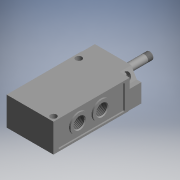
# Autodesk Inventor part: 6211 MFH-5-1/4
Saved by Autodesk Inventor 2017.3 (Build 213256000, 256)
## iProperties
Part Number: 6211 MFH-5-1/4
Material: Generic
Catalog Web Link: www.cadenas.de
Description: MFH-Solenoid valve
Vendor: FESTO
Document SubType Name: Modeling
Designer: partserver
Manufacturer: FESTO
Mass: 290 g
Surface Area: 238.767 cm^2
Volume: 130.921 cm^3
Density: 1 g/cm^3
Appearance: PSOLRGB-175-175-175
Category: PARTsolutions
Company: FESTO
Title: 6211 MFH-5-1/4
Author: Cadenas PARTsolutions
Comments: Solenoid valve
PSOL_IDENT_0: {$CADENAS_DATA\23d-libs\festo\parts\m\mfh\mfh.prj},166 {VTYP=3D},{NB=6211 MFH-5-1/4},{LINA=6211 MFH-
PSOL_IDENT_1: 5-1/4},{NN=MFH},{DATE=30.03.2021 15:09:58},{GEOMDATE=15.12.2020 07:36:11},{VERSION=},{LINEID=180},{W
PSOL_IDENT_2: BVAR=},{WBNUMERIC=}  {NB=6211 MFH-5-1/4},{LINA=6211 MFH-5-1/4},{KT=DUMMY},{TNR=6211},{TYP=MFH-5-1/4}
PSOL_IDENT_3: ,{INFO=},{S=0.000},{VERS=6.000},{AW=0.000},{A=30.000},{A1=49.600},{A2=14.000},{A3=12.500},{A4=19.600
PSOL_IDENT_4: },{A5=12.000},{A6=20.000},{A7=28.000},{A8=30.000},{A9=7.820},{A10=13.700},{A11=0.000},{A12=0.000},{A
PSOL_IDENT_5: 13=0.000},{A14=0.000},{A15=0.000},{A16=0.000},{A17=0.000},{L01=80.000},{EX=0.000},{EX1=0.000},{EX2=0
PSOL_IDENT_6: .000},{EX3=0.000},{EX4=0.000},{EX5=0.000},{EX6=0.000},{EXW=0.000},{L0=0.000},{L03=0.000},{B0=0.000},
PSOL_IDENT_7: {B=0.000},{B1=30.400},{B2=0.000},{B3=5.000},{B4=4.000},{B5=0.000},{B6=0.000},{B7=0.000},{B8=0.000},{
PSOL_IDENT_8: B9=0.000},{D1=G1/4},{D1P=13.157},{KDR1=11.445},{D2=M5},{D2P=5.000},{KDRD2=4.134},{D3=6.500},{D3P=0.0
PSOL_IDENT_9: 00},{KDRD3=0.000},{D4=0.000},{D5=0.000},{D6=0.000},{H1=128.000},{H2=143.000},{H3=12.000},{H4=24.000}
PSOL_IDENT_10: ,{H5=28.000},{H6=9.500},{H7=128.000},{H8=94.000},{H9=8.000},{H10=0.000},{H11=0.000},{H12=0.000},{H13=
PSOL_IDENT_11: 0.000},{H14=0.000},{H15=0.000},{H16=0.000},{H17=0.000},{H18=0.000},{H19=0.000},{H20=0.000},{H21=0.00
PSOL_IDENT_12: 0},{H22=0.000},{H23=0.000},{H24=0.000},{H25=0.000},{HR1=5.000},{HR2=72.000},{HR3=0.000},{HR4=0.000},
PSOL_IDENT_13: {L21=40.000},{K=0.000},{L1=50.000},{L2=74.000},{L3=0.000},{L4=0.000},{L5=0.000},{L6=0.000},{L8=0.000
PSOL_IDENT_14: },{L9=0.000},{L10=0.000},{L11=0.000},{L12=0.000},{PSTOL=0.1},{ZZZ=0.000},{V=0.000},{B00=0.000},{B01=
PSOL_IDENT_15: 0.000},{B02=0.000},{B03=0.000},{L02=0.000},{CNSMASSEXACT=0.290},{L7=MIN},{EOLDATE=}
NB: 6211 MFH-5-1/4
NN: MFH
NT: Solenoid valve
NBSYN: $TNR. $TYP.
LINA: 6211 MFH-5-1/4
CATALOG: Festo
OFFICIAL_STANDARD_NUMBERS: ISO 1, ISO 2, ISO 3, ISO 4
TNR: 6211
TYP: MFH-5-1/4
B: 0
B1: 30.4
B2: 0
B3: 5
B4: 4
B5: 0
B6: 0
B7: 0
B8: 0
B9: 0
D1: G1/4
D2: M5
D3: 6.5
D4: 0
D5: 0
D6: 0
H1: 128
H2: 143
H3: 12
H4: 24
H5: 28
H6: 9.5
H7: 128
H8: 94
H9: 8
H10: 0
H11: 0
H12: 0
H13: 0
H14: 0
H15: 0
H16: 0
H17: 0
H18: 0
H19: 0
H20: 0
H21: 0
H22: 0
H23: 0
H24: 0
H25: 0
HR1: 5
HR2: 72
HR3: 0
HR4: 0
L21: 40
L1: 50
L2: 74
L3: 0
L4: 0
L5: 0
L6: 0
L8: 0
L9: 0
L10: 0
L11: 0
L12: 0
CNSMASSEXACT: 0.29
SUPPLIER: FESTO
ARTICLENO: 6211 MFH-5-1/4
BOMINFO: 6211 MFH-5-1/4
CREATOR: CADENAS GmbH
Autodesk Inventor part; units mm, degrees
ref_plane "YZ Plane" through (0, 0, 0) normal (1, 0, 0) x (0, 1, 0)
ref_plane "XZ Plane" through (0, 0, 0) normal (0, 1, 0) x (-1, 0, 0)
ref_plane "XY Plane" through (0, 0, 0) normal (0, 0, 1) x (1, 0, 0)
sketch "Skizze_1" plane through (0, 0, 0) normal (0, 0, 1) x (1, 0, 0)
  line L0 (-25, 94) -> (-25, 0)
  line L1 (-25, 0) -> (25, 0)
  line L2 (25, 0) -> (25, 94)
  line L3 (25, 94) -> (-25, 94)
  constraints: 8 end point
extrude "Extrusion1" add sketch "Skizze_1" along normal mid plane 30.4
sketch "Sketch_1" plane through (0, 94, 0) normal (0, 1, 0) x (1, 0, 0)
  line L0 (-34.8, -25) -> (34.8, -25)
  line L1 (34.8, -25) -> (34.8, 25)
  line L2 (34.8, 25) -> (-34.8, 25)
  line L3 (-34.8, 25) -> (-34.8, -25)
  line L4 (-24.8, -15) -> (24.8, -15)
  line L5 (24.8, -15) -> (24.8, 15)
  line L6 (24.8, 15) -> (-24.8, 15)
  line L7 (-24.8, 15) -> (-24.8, -15)
  constraints: 16 end point
extrude "Extrusion2" cut sketch "Sketch_1" against normal blind 14
sketch "Sketch_9" plane through (0, 94, 0) normal (0, 1, 0) x (1, 0, 0)
  line L0 (-24.8, 4.6077) -> (-19.9719, 4.6077)
  line L1 (-19.9719, 4.6077) -> (-13.9719, 15)
  line L2 (-13.9719, 15) -> (-24.8, 15)
  line L3 (-24.8, 15) -> (-24.8, 4.6077)
  constraints: 8 end point
extrude "Extrusion3" cut sketch "Sketch_9" against normal blind 12.5
sketch "Sketch_10" plane through (0, 0, 10) normal (0, 0, 1) x (1, 0, 0)
  line L0 (-14, 92.8708) -> (-14, 94)
  line L1 (-14, 94) -> (-10.3, 94)
  line L2 (-10.3, 94) -> (-10.3, 89.4)
  line L3 (-10.3, 89.4) -> (-10.5, 89.4)
  line L4 (-10.5, 89.4) -> (-10.5, 92.9)
  arc A0 (-10.5, 92.9) -> (-11, 93.4) centre (-11, 92.9) ccw
  line L5 (-11, 93.4) -> (-12.025, 93.4)
  line L6 (-12.025, 93.4) -> (-14, 92.8708)
  line L7 (-14, 92.8708) -> (-14, 94)
  constraints: 16 end point, 2 point on circle, 1 centre point
revolve "Revolution1" cut sketch "Sketch_10" angle 360 about axis through (-14, 92.8708, 10) along (0, -1, 0)
sketch "Sketch_11" plane through (0, 0, -10) normal (0, 0, 1) x (1, 0, 0)
  line L0 (14, 92.8708) -> (14, 94)
  line L1 (14, 94) -> (17.7, 94)
  line L2 (17.7, 94) -> (17.7, 89.4)
  line L3 (17.7, 89.4) -> (17.5, 89.4)
  line L4 (17.5, 89.4) -> (17.5, 92.9)
  arc A0 (17.5, 92.9) -> (17, 93.4) centre (17, 92.9) ccw
  line L5 (17, 93.4) -> (15.975, 93.4)
  line L6 (15.975, 93.4) -> (14, 92.8708)
  line L7 (14, 92.8708) -> (14, 94)
  constraints: 16 end point, 2 point on circle, 1 centre point
revolve "Revolution2" cut sketch "Sketch_11" angle 360 about axis through (14, 92.8708, -10) along (0, -1, 0)
sketch "Sketch_12" plane through (0, 94, 0) normal (0, 1, 0) x (1, 0, 0)
  arc A0 (-15.1708, -8.8679) -> (-15.5658, -9.5521) centre (-15.3683, -9.21) ccw
  line L0 (-15.5658, -9.5521) -> (-15.54, -9.567)
  arc A1 (-15.54, -10.433) -> (-15.54, -9.567) centre (-15.79, -10) ccw
  line L1 (-15.54, -10.433) -> (-15.5658, -10.4479)
  arc A2 (-15.5658, -10.4479) -> (-15.1708, -11.1321) centre (-15.3683, -10.79) ccw
  line L2 (-15.1708, -11.1321) -> (-15.145, -11.1172)
  arc A3 (-14.395, -11.5502) -> (-15.145, -11.1172) centre (-14.895, -11.5502) ccw
  line L3 (-14.395, -11.5502) -> (-14.395, -11.58)
  arc A4 (-14.395, -11.58) -> (-13.605, -11.58) centre (-14, -11.58) ccw
  line L4 (-13.605, -11.58) -> (-13.605, -11.5502)
  arc A5 (-12.855, -11.1172) -> (-13.605, -11.5502) centre (-13.105, -11.5502) ccw
  line L5 (-12.855, -11.1172) -> (-12.8292, -11.1321)
  arc A6 (-12.8292, -11.1321) -> (-12.4342, -10.4479) centre (-12.6317, -10.79) ccw
  line L6 (-12.4342, -10.4479) -> (-12.46, -10.433)
  arc A7 (-12.46, -9.567) -> (-12.46, -10.433) centre (-12.21, -10) ccw
  line L7 (-12.46, -9.567) -> (-12.4342, -9.5521)
  arc A8 (-12.4342, -9.5521) -> (-12.8292, -8.8679) centre (-12.6317, -9.21) ccw
  line L8 (-12.8292, -8.8679) -> (-12.855, -8.8828)
  arc A9 (-13.605, -8.4498) -> (-12.855, -8.8828) centre (-13.105, -8.4498) ccw
  line L9 (-13.605, -8.4498) -> (-13.605, -8.42)
  arc A10 (-13.605, -8.42) -> (-14.395, -8.42) centre (-14, -8.42) ccw
  line L10 (-14.395, -8.42) -> (-14.395, -8.4498)
  arc A11 (-15.145, -8.8828) -> (-14.395, -8.4498) centre (-14.895, -8.4498) ccw
  line L11 (-15.145, -8.8828) -> (-15.1708, -8.8679)
  constraints: 24 end point, 24 point on circle, 12 centre point
extrude "Extrusion4" cut sketch "Sketch_12" against normal blind 2.4
sketch "Sketch_13" plane through (0, 94, 0) normal (0, 1, 0) x (1, 0, 0)
  arc A0 (12.4342, 9.5521) -> (12.8292, 8.8679) centre (12.6317, 9.21) ccw
  line L0 (12.8292, 8.8679) -> (12.855, 8.8828)
  arc A1 (13.605, 8.4498) -> (12.855, 8.8828) centre (13.105, 8.4498) ccw
  line L1 (13.605, 8.4498) -> (13.605, 8.42)
  arc A2 (13.605, 8.42) -> (14.395, 8.42) centre (14, 8.42) ccw
  line L2 (14.395, 8.42) -> (14.395, 8.4498)
  arc A3 (15.145, 8.8828) -> (14.395, 8.4498) centre (14.895, 8.4498) ccw
  line L3 (15.145, 8.8828) -> (15.1708, 8.8679)
  arc A4 (15.1708, 8.8679) -> (15.5658, 9.5521) centre (15.3683, 9.21) ccw
  line L4 (15.5658, 9.5521) -> (15.54, 9.567)
  arc A5 (15.54, 10.433) -> (15.54, 9.567) centre (15.79, 10) ccw
  line L5 (15.54, 10.433) -> (15.5658, 10.4479)
  arc A6 (15.5658, 10.4479) -> (15.1708, 11.1321) centre (15.3683, 10.79) ccw
  line L6 (15.1708, 11.1321) -> (15.145, 11.1172)
  arc A7 (14.395, 11.5502) -> (15.145, 11.1172) centre (14.895, 11.5502) ccw
  line L7 (14.395, 11.5502) -> (14.395, 11.58)
  arc A8 (14.395, 11.58) -> (13.605, 11.58) centre (14, 11.58) ccw
  line L8 (13.605, 11.58) -> (13.605, 11.5502)
  arc A9 (12.855, 11.1172) -> (13.605, 11.5502) centre (13.105, 11.5502) ccw
  line L9 (12.855, 11.1172) -> (12.8292, 11.1321)
  arc A10 (12.8292, 11.1321) -> (12.4342, 10.4479) centre (12.6317, 10.79) ccw
  line L10 (12.4342, 10.4479) -> (12.46, 10.433)
  arc A11 (12.46, 9.567) -> (12.46, 10.433) centre (12.21, 10) ccw
  line L11 (12.46, 9.567) -> (12.4342, 9.5521)
  constraints: 24 end point, 24 point on circle, 12 centre point
extrude "Extrusion5" cut sketch "Sketch_13" against normal blind 2.4
sketch "Skizze_3" plane through (0, 0, 0) normal (0, 0, 1) x (1, 0, 0)
  circle A0 centre (-20, 5) radius 3.25
  constraints: 1 centre point
extrude "Extrusion6" cut sketch "Skizze_3" along normal mid plane 60.8
sketch "Skizze_13" plane through (0, 0, 0) normal (0, 0, 1) x (1, 0, 0)
  circle A0 centre (20, 72) radius 3.25
  constraints: 1 centre point
extrude "Extrusion7" cut sketch "Skizze_13" along normal mid plane 60.8
sketch "Skizze_7" plane through (-25, 0, -15.2) normal (-1, 0, 0) x (0, 0, 1)
  line L0 (2.0064, 52) -> (2.0064, 6.5664)
  arc A0 (2.0064, 6.5664) -> (3.0096, 5.5632) centre (3.0096, 6.5664) ccw
  line L1 (3.0096, 5.5632) -> (27.3904, 5.5632)
  arc A1 (27.3904, 5.5632) -> (28.3936, 6.5664) centre (27.3904, 6.5664) ccw
  line L2 (28.3936, 6.5664) -> (28.3936, 52)
  line L3 (28.3936, 52) -> (2.0064, 52)
  constraints: 8 end point, 4 point on circle, 2 centre point
extrude "Extrusion8" cut sketch "Skizze_7" along normal mid plane 3
sketch "Sketch_3" plane through (-25, 0, -15.2) normal (-1, 0, 0) x (0, 0, 1)
  line L0 (2.0064, 74.9904) -> (2.0064, 52)
  line L1 (2.0064, 52) -> (28.3936, 52)
  line L2 (28.3936, 52) -> (28.3936, 74.9904)
  arc A0 (28.3936, 74.9904) -> (27.3904, 75.9936) centre (27.3904, 74.9904) ccw
  line L3 (27.3904, 75.9936) -> (3.0096, 75.9936)
  arc A1 (3.0096, 75.9936) -> (2.0064, 74.9904) centre (3.0096, 74.9904) ccw
  constraints: 8 end point, 4 point on circle, 2 centre point
extrude "Extrusion9" cut sketch "Sketch_3" against normal blind 1.5
sketch "Skizze_15" plane through (-25, 0, -15.2) normal (-1, 0, 0) x (0, 0, 1)
  circle A0 centre (15.2, 52) radius 9.8678
  constraints: 1 centre point
extrude "Extrusion10" add sketch "Skizze_15" against normal blind 1.5
sketch "Skizze_6" plane through (0, 0, 0) normal (0, 0, 1) x (1, 0, 0)
  line L0 (-12.5, 52) -> (-25, 52)
  line L1 (-25, 52) -> (-25, 58.5785)
  line L2 (-25, 58.5785) -> (-24.144, 57.7225)
  line L3 (-24.144, 57.7225) -> (-12.5, 57.7225)
  line L4 (-12.5, 57.7225) -> (-12.5, 52)
  line L5 (-12.5, 52) -> (-25, 52)
  constraints: 12 end point
revolve "Revolution3" cut sketch "Skizze_6" angle 360 about axis through (-12.5, 52, 0) along (1, 0, 0)
thread "Thread1" size "G13.157x1.337" designation "G 1/4" standard "ISO Pipe Threads" full length
sketch "Skizze_16" plane through (-25, 0, 15.2) normal (-1, 0, 0) x (0, 1, 0)
  circle A0 centre (28, 15.2) radius 9.8678
  constraints: 1 centre point
extrude "Extrusion11" add sketch "Skizze_16" against normal blind 2
sketch "Skizze_8" plane through (0, 0, 0) normal (0, 0, 1) x (1, 0, 0)
  line L0 (-12.5, 28) -> (-25, 28)
  line L1 (-25, 28) -> (-25, 34.5785)
  line L2 (-25, 34.5785) -> (-24.144, 33.7225)
  line L3 (-24.144, 33.7225) -> (-12.5, 33.7225)
  line L4 (-12.5, 33.7225) -> (-12.5, 28)
  line L5 (-12.5, 28) -> (-25, 28)
  constraints: 12 end point
revolve "Revolution4" cut sketch "Skizze_8" angle 360 about axis through (-12.5, 28, 0) along (1, 0, 0)
thread "Thread2" size "G13.157x1.337" designation "G 1/4" standard "ISO Pipe Threads" full length
sketch "Skizze_17" plane through (25, 0, 15.2) normal (1, 0, 0) x (0, 0, -1)
  line L0 (1.824, 75.1728) -> (1.824, 2.8272)
  arc A0 (1.824, 2.8272) -> (2.8272, 1.824) centre (2.8272, 2.8272) ccw
  line L1 (2.8272, 1.824) -> (27.5728, 1.824)
  arc A1 (27.5728, 1.824) -> (28.576, 2.8272) centre (27.5728, 2.8272) ccw
  line L2 (28.576, 2.8272) -> (28.576, 75.1728)
  arc A2 (28.576, 75.1728) -> (27.5728, 76.176) centre (27.5728, 75.1728) ccw
  line L3 (27.5728, 76.176) -> (2.8272, 76.176)
  arc A3 (2.8272, 76.176) -> (1.824, 75.1728) centre (2.8272, 75.1728) ccw
  constraints: 8 end point, 8 point on circle, 4 centre point
extrude "Extrusion12" cut sketch "Skizze_17" along normal mid plane 3
sketch "Skizze_18" plane through (25, 0, 15.2) normal (1, 0, 0) x (0, 0, -1)
  circle A0 centre (15.2, 12) radius 9.8678
  constraints: 1 centre point
extrude "Extrusion13" add sketch "Skizze_18" against normal blind 2
sketch "Skizze_19" plane through (25, 0, 15.2) normal (1, 0, 0) x (0, 0, -1)
  circle A0 centre (10.2, 36) radius 9.8678
  constraints: 1 centre point
extrude "Extrusion14" add sketch "Skizze_19" against normal blind 2.05
sketch "Skizze_20" plane through (25, 0, 15.2) normal (1, 0, 0) x (0, 0, -1)
  circle A0 centre (15.2, 60) radius 9.8678
  constraints: 1 centre point
extrude "Extrusion15" add sketch "Skizze_20" against normal blind 2
sketch "Skizze_5" plane through (0, 0, 0) normal (0, 0, 1) x (1, 0, 0)
  line L0 (25, 60) -> (12.5, 60)
  line L1 (12.5, 60) -> (12.5, 65.7225)
  line L2 (12.5, 65.7225) -> (24.144, 65.7225)
  line L3 (24.144, 65.7225) -> (25, 66.5785)
  line L4 (25, 66.5785) -> (25, 60)
  line L5 (25, 60) -> (12.5, 60)
  constraints: 12 end point
revolve "Revolution5" cut sketch "Skizze_5" angle 360 about axis through (25, 60, 0) along (1, 0, 0)
thread "Thread3" size "G13.157x1.337" designation "G 1/4" standard "ISO Pipe Threads" full length
sketch "Skizze_10" plane through (0, 0, 0) normal (0, 0, 1) x (1, 0, 0)
  line L0 (25, 12) -> (12.5, 12)
  line L1 (12.5, 12) -> (12.5, 17.7225)
  line L2 (12.5, 17.7225) -> (24.144, 17.7225)
  line L3 (24.144, 17.7225) -> (25, 18.5785)
  line L4 (25, 18.5785) -> (25, 12)
  line L5 (25, 12) -> (12.5, 12)
  constraints: 12 end point
revolve "Revolution6" cut sketch "Skizze_10" angle 360 about axis through (25, 12, 0) along (1, 0, 0)
thread "Thread4" size "G13.157x1.337" designation "G 1/4" standard "ISO Pipe Threads" full length
sketch "Skizze_9" plane through (0, 0, 5) normal (0, 0, 1) x (1, 0, 0)
  line L0 (25, 36) -> (12.5, 36)
  line L1 (12.5, 36) -> (12.5, 41.7225)
  line L2 (12.5, 41.7225) -> (24.144, 41.7225)
  line L3 (24.144, 41.7225) -> (25, 42.5785)
  line L4 (25, 42.5785) -> (25, 36)
  line L5 (25, 36) -> (12.5, 36)
  constraints: 12 end point
revolve "Revolution7" cut sketch "Skizze_9" angle 360 about axis through (25, 36, 5) along (1, 0, 0)
thread "Thread5" size "G13.157x1.337" designation "G 1/4" standard "ISO Pipe Threads" full length
sketch "Skizze_24" plane through (0, 94, 0) normal (0, 1, 0) x (1, 0, 0)
  line L0 (-6.5, -3.7528) -> (0, -7.5056)
  line L1 (0, -7.5056) -> (6.5, -3.7528)
  line L2 (6.5, -3.7528) -> (6.5, 3.7528)
  line L3 (6.5, 3.7528) -> (0, 7.5056)
  line L4 (0, 7.5056) -> (-6.5, 3.7528)
  line L5 (-6.5, 3.7528) -> (-6.5, -3.7528)
  constraints: 12 end point
extrude "Extrusion16" add sketch "Skizze_24" along normal blind 2
sketch "Skizze_25" plane through (0, 0, 0) normal (0, 0, 1) x (1, 0, 0)
  line L0 (0, 88) -> (0, 128)
  line L1 (0, 128) -> (3.54, 128)
  line L2 (3.54, 128) -> (4, 127.54)
  line L3 (4, 127.54) -> (4, 88)
  line L4 (4, 88) -> (0, 88)
  line L5 (0, 88) -> (0, 128)
  constraints: 12 end point
revolve "Revolution8" add sketch "Skizze_25" angle 360 about axis through (0, 88, 0) along (0, -1, 0)
thread "Thread6" size "M8x0.75" class "6g" standard "ISO Metric profile" length 5.54
sketch "Sketch30" plane through (0, 128, 0) normal (0, 1, 0) x (1, 0, 0)
  point P0 (0, 0)
hole "Hole1" at (0, 128, 0) direction (0, -1, 0) diameter 4.134 depth 6 tip angle 120 countersink diameter 5 countersink angle 90 thread size "M5x0.8" class "6H" standard "ISO Metric profile"
sketch "Sketch_14" plane through (0, 0, 0) normal (0.5, 0, -0.8660254) x (-0.8660254, 0, -0.5)
  line L0 (19.6, 86.18) -> (16.2, 86.18)
  line L1 (16.2, 86.18) -> (16.2, 89.52)
  line L2 (16.2, 89.52) -> (15.8, 89.92)
  line L3 (15.8, 89.92) -> (15.7382, 89.92)
  line L4 (15.7382, 89.92) -> (19.6, 90.28)
  line L5 (19.6, 90.28) -> (19.6, 86.18)
  line L6 (19.6, 86.18) -> (16.2, 86.18)
  constraints: 14 end point
revolve "Revolution9" cut sketch "Sketch_14" angle 360 about axis through (-16.9741, 86.18, -9.8) along (-0.8660254, 0, -0.5)
sketch "Sketch_15" plane through (0, 0, 0) normal (0.5, 0, -0.8660254) x (-0.8660254, 0, -0.5)
  line L0 (14.8, 82.44) -> (16.2, 82.44)
  line L1 (16.2, 82.44) -> (16.2, 89.92)
  line L2 (16.2, 89.92) -> (14.8, 89.92)
  line L3 (14.8, 89.92) -> (14.8, 82.44)
  constraints: 8 end point
extrude "Extrusion17" cut sketch "Sketch_15" along normal mid plane 1
sketch "Sketch_27" plane through (0, 0, 0) normal (0.5, 0, -0.8660254) x (-0.8660254, 0, -0.5)
  line L0 (19.6, 86.18) -> (0, 86.18)
  line L1 (15.7382, 90.92) -> (15.7382, 89.92)
  line L2 (15.7382, 89.92) -> (19.6, 90.28)
  line L3 (19.6, 90.28) -> (19.6, 90.92)
  line L4 (19.6, 90.92) -> (15.7382, 90.92)
  constraints: 10 end point
revolve "Revolution10" add sketch "Sketch_27" angle 360 about axis through (-16.9741, 86.18, -9.8) along (-0.8660254, 0, -0.5)
ref_plane "PART1_XY" through (0, 0, 0) normal (0, 1, 0) x (1, 0, 0)
ref_plane "PART1_YZ" through (0, 0, 0) normal (1, 0, 0) x (0, 0, -1)
ref_plane "PART1_ZX" through (0, 0, 0) normal (0, 0, -1) x (0, 1, 0)
body "Solid1"
